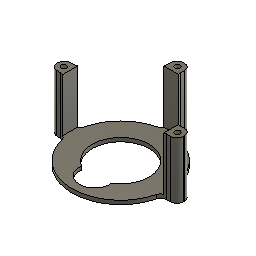
Bottom (Autodesk Fusion 360 design; units mm, degrees)
Autodesk Fusion 360 part; units mm, degrees
sketch "Sketch1" plane through (0, 0, 0) normal (0, 1, 0) x (1, 0, 0)
  circle A0 centre (0, 0) radius 22.5
  circle A1 centre (0, 0) radius 38.5
  line L0 (0, 0) -> (0, 100.2102) construction
  line L1 (0, 0) -> (100.2102, 0) construction
  line L2 (38.1051, 5.5) -> (50.1051, 5.5)
  line L3 (50.1051, 5.5) -> (50.1051, -5.5)
  line L4 (50.1051, -5.5) -> (38.1051, -5.5)
  line L5 (-50.1051, -5.5) -> (-38.1051, -5.5)
  line L6 (-38.1051, 5.5) -> (-50.1051, 5.5)
  line L7 (-50.1051, 5.5) -> (-50.1051, -5.5)
  line L8 (-5.5, 50.1051) -> (5.5, 50.1051)
  line L9 (5.5, 50.1051) -> (5.5, 38.1051)
  line L10 (-5.5, 38.1051) -> (-5.5, 50.1051)
  line L11 (0, 0) -> (0, -42.9261) construction
  circle A2 centre (0, -20.6548) radius 12
  dimension "d1" = 45
  dimension "d2" = 16
  dimension "d4" = 11
  dimension "d5" = 12
  dimension "d8" = 24
  constraint coincident A0.centre A1.centre
  constraint vertical L0
  constraint perpendicular L0 L1
  constraint horizontal L2
  constraint vertical L3
  constraint horizontal L4
  constraint midpoint L1 L3
  constraint coincident A1 L2.start
  constraint symmetric L0 L2.end L6.end
  constraint symmetric L0 L3.end L5.start
  constraint symmetric L0 L4.end L5.end
  constraint symmetric L0 L2.start L6.start
  constraint horizontal L8
  constraint vertical L9
  constraint vertical L10
  constraint midpoint L0 L8
  constraint coincident A1 L10.start
  constraint equal L7 L8
  constraint equal L6 L9
  constraint perpendicular L1 L11
  constraint coincident L11 A2.centre
  measures "d1" diameter of A0
  measures "d2" distance of A0 A1
  measures "d4" distance of L2.end L3.end
  measures "d5" distance of L2.end L2.start
  measures "d8" diameter of A2
extrude "Extrude1" add sketch "Sketch1" along normal blind 3 makes body 1 in component "Body"
ref_plane "WorkPlane1" through (0, 3, -5.8026) normal (0, 1, 0) x (1, 0, 0)
sketch "Sketch2" plane through (0, 3, -5.8026) normal (0, 1, 0) x (1, 0, 0)
  line L0 (-5.5, 44.3026) -> (5.5, 44.3026)
  line L1 (5.5, 44.3026) -> (5.5, 34.3026)
  line L2 (5.5, 34.3026) -> (-5.5, 34.3026)
  line L3 (-5.5, 34.3026) -> (-5.5, 44.3026)
  line L4 (-50.1051, -0.3026) -> (-40.1051, -0.3026)
  line L5 (-40.1051, -0.3026) -> (-40.1051, -11.3026)
  line L6 (-40.1051, -11.3026) -> (-50.1051, -11.3026)
  line L7 (-50.1051, -11.3026) -> (-50.1051, -0.3026)
  line L8 (0, 0) -> (0, 69.9083) construction
  line L9 (50.1051, -11.3026) -> (50.1051, -0.3026)
  line L10 (40.1051, -0.3026) -> (40.1051, -11.3026)
  line L11 (40.1051, -11.3026) -> (50.1051, -11.3026)
  line L12 (50.1051, -0.3026) -> (40.1051, -0.3026)
  point P0 (-5.5, 44.3026)
  point P1 (5.5, 44.3026)
  point P2 (-50.1051, -11.3026)
  point P3 (-50.1051, -0.3026)
  point P4 (50.1051, -0.3026)
  point P5 (50.1051, -11.3026)
  dimension "d10" = 10
  constraint horizontal L0
  constraint vertical L1
  constraint horizontal L2
  constraint vertical L3
  constraint coincident P0 L0.start
  constraint coincident P1 L0.end
  constraint horizontal L4
  constraint vertical L5
  constraint horizontal L6
  constraint vertical L7
  constraint coincident P2 L6.end
  constraint coincident P3 L4.start
  constraint equal L1 L4
  constraint coincident L8.start origin
  constraint perpendicular L0 L8
  constraint symmetric P3 L8 P4
  constraint symmetric L4.end L8 L10.start
  constraint symmetric L5.end L8 L10.end
  constraint symmetric P2 L8 P5
  measures "d10" distance of P1 L1.end
extrude "Extrude2" add sketch "Sketch2" along normal blind 42 bodies 1 in component "Body"
ref_plane "WorkPlane2" through (0, 45, -45.1051) normal (0, 1, 0) x (0, 0, 1)
sketch "Sketch3" plane through (0, 45, -45.1051) normal (0, 1, 0) x (1, 0, 0)
  circle A0 centre (0, 0) radius 2.1
  line L0 (-45.1051, -39.6051) -> (-45.1051, -50.6051) construction
  line L1 (-50.1051, -45.1051) -> (-40.1051, -45.1051) construction
  line L2 (-40.1051, -39.6051) -> (-50.1051, -39.6051) construction
  line L3 (-50.1051, -50.6051) -> (-40.1051, -50.6051) construction
  line L4 (-50.1051, -39.6051) -> (-50.1051, -50.6051) construction
  line L5 (-40.1051, -50.6051) -> (-40.1051, -39.6051) construction
  circle A1 centre (-45.1051, -45.1051) radius 2.1
  line L6 (0, 33.7384) -> (0, -58.8388)
  circle A2 centre (45.1051, -45.1051) radius 2.1
  dimension "d14" = 4.2
  constraint coincident A0.centre origin
  constraint vertical L0
  constraint horizontal L1
  constraint midpoint L0 L1
  constraint coincident L0.start L2
  constraint coincident L0.end L3
  constraint coincident L1.start L4
  constraint coincident L1.end L5
  constraint midpoint L1 A1.centre
  constraint equal A0 A1
  constraint vertical L6
  constraint symmetric A1 L6 A2
  measures "d14" diameter of A0
extrude "Extrude3" cut sketch "Sketch3" against normal up to surface (45 mm away) bodies 1 in component "Body"
ref_plane "WorkPlane3" through (0, 45, -45.1051) normal (0, 1, 0) x (0, 0, 1)
sketch "Sketch4" plane through (0, 45, -45.1051) normal (0, 1, 0) x (1, 0, 0)
  circle A0 centre (0, -45.1051) radius 38.5
  arc A1 (-5.5, -7) -> (-38.1051, -39.6051) centre (0, -45.1051) ccw
  line L0 (-5.5, 5) -> (5.5, 5)
  line L1 (5.5, 5) -> (5.5, -7)
  line L2 (-5.5, -7) -> (-5.5, 5)
  line L3 (-50.1051, -39.6051) -> (-38.1051, -39.6051)
  line L4 (-38.1051, -50.6051) -> (-50.1051, -50.6051)
  line L5 (-50.1051, -50.6051) -> (-50.1051, -39.6051)
  line L6 (0, -45.1051) -> (0, 55.1083) construction
  circle A2 centre (-45.1051, -45.1051) radius 2.1
  circle A3 centre (-45.1051, -45.1051) radius 2.1
  circle A4 centre (0, 0) radius 2.1
  circle A5 centre (45.1051, -45.1051) radius 2.1
  line L7 (50.1051, -39.6051) -> (38.1051, -39.6051)
  circle A6 centre (45.1051, -45.1051) radius 2.1
  line L8 (38.1051, -50.6051) -> (50.1051, -50.6051)
  line L9 (50.1051, -50.6051) -> (50.1051, -39.6051)
  circle A7 centre (0, -45.1051) radius 15.5
  circle A8 centre (0, -45.1051) radius 17.5
  circle A9 centre (0, 0) radius 2.1
  point P0 (-5.5, 5)
  point P1 (5.5, 5)
  point P2 (-50.1051, -39.6051)
  point P3 (-50.1051, -50.6051)
  point P4 (50.1051, -50.6051)
  point P5 (38.1051, -39.6051)
  point P6 (50.1051, -39.6051)
  dimension "d28" = 2
  dimension "d29" = 35
  constraint equal A0 A1
  constraint tangent A0 A1
  constraint horizontal L0
  constraint vertical L1
  constraint vertical L2
  constraint coincident P0 L0.start
  constraint coincident P1 L0.end
  constraint coincident A0 L1.end
  constraint horizontal L3
  constraint horizontal L4
  constraint vertical L5
  constraint coincident P2 L3.start
  constraint coincident P3 L4.end
  constraint coincident A0 L4.start
  constraint coincident A0.centre A1.centre
  constraint vertical L6
  constraint equal A2 A3
  constraint tangent A2 A3
  constraint symmetric A1.end L6 P5
  constraint symmetric P2 L6 P6
  constraint symmetric L4.start L6 L8.start
  constraint symmetric P3 L6 P4
  constraint symmetric L6 A2 A5
  constraint symmetric L6 A3 A6
  constraint concentric A1 A7
  constraint concentric A1 A8
  constraint concentric A4 A9
  constraint equal A4 A9
  measures "d28" distance of A7 A8
  measures "d29" diameter of A8
extrude "Extrude2'" add sketch "Sketch4" along normal blind 50 separate body contours A8 makes body 2
extrude "Extrude1'" add sketch "Sketch4" along normal blind 3 contours A0 A1 | A0 L7 L8 L9 | A0 L0 L1 L2 | A0 L3 L4 L5 bodies 2
copy_body "Body->Comp1" bodies 2 removing the originals makes body 3 in component "Top"
fillet "Fillet1" radius 5 6 edges at (50.1051, 46.5, 5.5) (50.1051, 46.5, -5.5) (-5.5, 46.5, -50.1051) (5.5, 46.5, -50.1051) (-50.1051, 46.5, -5.5) (-50.1051, 46.5, 5.5) on bodies 3 in component "Top"
fillet "Fillet2" radius 5 6 edges at (-5.5, 22.5, -50.1051) (5.5, 22.5, -50.1051) (-50.1051, 22.5, -5.5) (-50.1051, 22.5, 5.5) (50.1051, 22.5, -5.5) (50.1051, 22.5, 5.5) on bodies 1 in component "Body"
fillet "Fillet2'" radius 5 1 edges at (-16.3157, 48, 6.3283) on bodies 3 in component "Top"
fillet "Fillet3" radius 5 6 edges at (38.1051, 1.5, 5.5) (38.1051, 1.5, -5.5) (5.5, 1.5, -38.1051) (-5.5, 1.5, -38.1051) (-38.1051, 1.5, -5.5) (-38.1051, 1.5, 5.5) on bodies 1 in component "Body"
fillet "Fillet3'" radius 5 6 edges at (38.1051, 46.5, -5.5) (38.1051, 46.5, 5.5) (5.5, 46.5, -38.1051) (-5.5, 46.5, -38.1051) (-38.1051, 46.5, -5.5) (-38.1051, 46.5, 5.5) on bodies 3 in component "Top"
component "Body" placed x (1, 0, 0) y (0, 1, 0) z (0, 0, 1) at (0, 0, 0)
component "Top" placed x (1, 0, 0) y (0, 1, 0) z (0, 0, 1) at (0, 0, 0)
